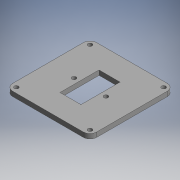
# Autodesk Inventor part: Part8
Saved by Autodesk Inventor 2019.2 (Build 232265000, 265)
## iProperties
Part Number: Part8
Material: Generic
Document SubType Name: Modeling
Designer: richard.girt
Mass: 6.06533 g
Surface Area: 52.0529 cm^2
Volume: 6.06533 cm^3
Density: 1 g/cm^3
Appearance: Default
Author: richard.girt
Autodesk Inventor part; units mm, degrees
ref_plane "YZ Plane" through (0, 0, 0) normal (1, 0, 0) x (0, 1, 0)
ref_plane "XZ Plane" through (0, 0, 0) normal (0, 1, 0) x (-1, 0, 0)
ref_plane "XY Plane" through (0, 0, 0) normal (0, 0, 1) x (1, 0, 0)
sketch "Sketch1" plane through (0, 0, 0) normal (0, 1, 0) x (-1, 0, 0)
  line L0 (-25, 25) -> (25, 25)
  line L1 (25, 25) -> (25, -25)
  line L2 (25, -25) -> (-25, -25)
  line L3 (-25, -25) -> (-25, 25)
  line L4 (-25, 25) -> (25, -25) construction
  line L5 (25, 25) -> (-25, -25) construction
  point P0 (0, 0)
  dimension "d0" = 50
  constraints: 12 end point, 2 midpoint, 2 parallel, 2 perpendicular, 1 horizontal
  measures "d0" distance of L2.end L0.start
extrude "Extrusion1" add sketch "Sketch1" along normal mid plane 2.8
sketch "Sketch2" plane through (0, 1.4, 0) normal (0, 1, 0) x (1, 0, 0)
  line L0 (-6.25, -11.625) -> (6.25, -11.625)
  line L1 (6.25, -11.625) -> (6.25, 11.625)
  line L2 (6.25, 11.625) -> (-6.25, 11.625)
  line L3 (-6.25, 11.625) -> (-6.25, -11.625)
  line L4 (-6.25, -11.625) -> (6.25, 11.625) construction
  line L5 (6.25, -11.625) -> (-6.25, 11.625) construction
  point P0 (0, 0)
  dimension "d3" = 12.5
  dimension "d4" = 23.25
  constraints: 12 end point, 2 midpoint, 2 parallel, 1 horizontal, 1 perpendicular
  measures "d3" distance of L1.end L2.end
  measures "d4" distance of L0.end L1.end
extrude "Extrusion2" cut sketch "Sketch2" against normal through all
sketch "Sketch3" plane through (0, 1.4, 0) normal (0, 1, 0) x (1, 0, 0)
  line L0 (6.25, 11.625) -> (6.25, -11.625) construction
  line L1 (6.25, -11.625) -> (-6.25, -11.625) construction
  line L2 (-6.25, -11.625) -> (-6.25, 11.625) construction
  line L3 (-6.25, 11.625) -> (6.25, 11.625) construction
  line L4 (-25, -25) -> (25, -25) construction
  line L5 (25, -25) -> (25, 25) construction
  line L6 (25, 25) -> (-25, 25) construction
  line L7 (-25, 25) -> (-25, -25) construction
  line L8 (-21.9203, 21.9203) -> (21.9203, 21.9203)
  line L9 (21.9203, 21.9203) -> (21.9203, -21.9203)
  line L10 (21.9203, -21.9203) -> (-21.9203, -21.9203)
  line L11 (-21.9203, -21.9203) -> (-21.9203, 21.9203)
  line L12 (-9.5, 14.875) -> (-9.5, -14.875)
  line L13 (-9.5, -14.875) -> (9.5, -14.875)
  line L14 (9.5, -14.875) -> (9.5, 14.875)
  line L15 (9.5, 14.875) -> (-9.5, 14.875)
  point P0 (0, 0)
  point P1 (-9.5, 0)
  point P2 (9.5, 0)
  dimension "d7" = 62
  dimension "d8" = 19
  constraints: 16 end point, 4 coincident, 2 midpoint, 6 other
  measures "d7" distance of point (-21.92, -21.92) point (21.92, 21.92)
  measures "d8" distance of L12.end L13.end
hole "Hole1" at (-21.9203, 1.4, -21.9203) at (21.9203, 1.4, -21.9203) at (21.9203, 1.4, 21.9203) at (-21.9203, 1.4, 21.9203) at (-9.5, 1.4, 0) at (9.5, 1.4, 0) direction (0, -1, 0) diameter 2.5 end through all
fillet "Fillet1" radius 4 4 edges at (-25, 0, -25) (25, 0, -25) (25, 0, 25) (-25, 0, 25)
body "Solid1"
